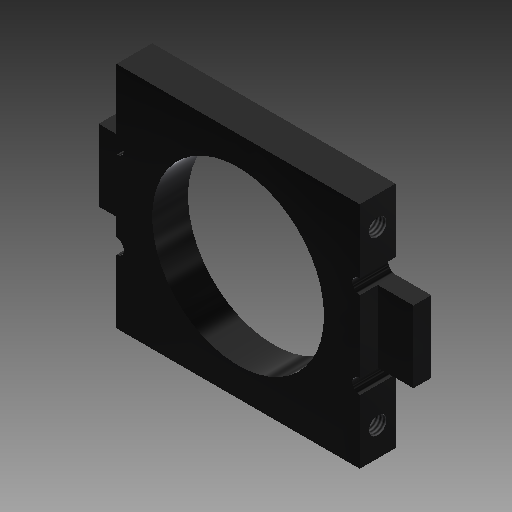
# Autodesk Inventor part: コックピット_2_サブフレーム_6
Saved by Autodesk Inventor 2018 (Build 220112000, 112)
## iProperties
Category: コックピット
Created: 2016-05-24
Part Number: コックピット_2_サブフレーム_6
Material: アセタール樹脂、黒
Document SubType Name: Modeling
Designer: hiroaki
Density: 1.425 g/cm^3
Appearance: 滑らか - 黒
Mass: 4.76795 g
Surface Area: 26.4558 cm^2
Volume: 3.34593 cm^3
Author: hiroaki
Autodesk Inventor part; units mm, degrees
ref_plane "YZ Plane" through (0, 0, 0) normal (1, 0, 0) x (0, 1, 0)
ref_plane "XZ Plane" through (0, 0, 0) normal (0, 1, 0) x (-1, 0, 0)
ref_plane "XY Plane" through (0, 0, 0) normal (0, 0, 1) x (1, 0, 0)
sketch "スケッチ1" plane through (0, 0, 0) normal (0, 0, 1) x (1, 0, 0)
  line L0 (-17, -16) -> (17, -16) construction
  line L1 (17, -16) -> (17, 16) construction
  line L2 (17, 16) -> (-17, 16) construction
  line L3 (-17, 16) -> (-17, -16) construction
  line L4 (-17, -16) -> (17, 16) construction
  line L5 (17, -16) -> (-17, 16) construction
  line L6 (-17, 7.1) -> (-17, 16)
  line L7 (-17, 16) -> (17, 16)
  line L8 (17, 16) -> (17, 7.1)
  line L9 (-17, 5) -> (-22, 5)
  line L10 (-22, 5) -> (-22, -5)
  line L11 (-22, -5) -> (-17, -5)
  line L12 (17, 5) -> (22, 5)
  line L13 (22, 5) -> (22, -5)
  line L14 (22, -5) -> (17, -5)
  line L15 (-17, -7.1) -> (-17, -16)
  line L16 (-17, -16) -> (17, -16)
  line L17 (17, -16) -> (17, -7.1)
  arc A0 (-17, 5) -> (-17, 7.1) centre (-17, 6.05) ccw
  arc A1 (-17, -7.1) -> (-17, -5) centre (-17, -6.05) ccw
  arc A2 (17, 7.1) -> (17, 5) centre (17, 6.05) ccw
  arc A3 (17, -5) -> (17, -7.1) centre (17, -6.05) ccw
  line L18 (0, 0) -> (-17, 0) construction
  line L19 (0, 0) -> (0, 16) construction
  dimension "d87" = 32
  dimension "d88" = 1.05
  dimension "d89" = 5
  dimension "d90" = 11
  dimension "d91" = 34
  constraints: 40 end point, 8 point on circle, 6 collinear, 6 perpendicular, 4 centre point, 4 horizontal, 4 midpoint, 4 point on line, 3 equal radius, 3 parallel, 3 symmetric about line, 2 tangent, 1 vertical, 3 other
  measures "d87" distance of L2.end L0.start
  measures "d88" radius of A0
  measures "d89" distance between parallel lines of L10 L3
  measures "d90" distance between parallel lines of L2 L9
  measures "d91" distance of L1.end L2.end
extrude "押し出し1" add sketch "スケッチ1" along normal blind 5
sketch "スケッチ2" plane through (0, 0, 5) normal (0, 0, 1) x (1, 0, 0)
  line L0 (-17, 16) -> (-17, 7.1) projected
  line L1 (17, 7.1) -> (17, 16) projected
  line L2 (-28.2886, 18.8938) -> (-17, 18.8938)
  line L3 (-17, 18.8938) -> (-17, -23.6662)
  line L4 (-17, -23.6662) -> (-28.2886, -23.6662)
  line L5 (-28.2886, -23.6662) -> (-28.2886, 18.8938)
  line L6 (17, 13.565) -> (34.37, 13.565)
  line L7 (34.37, 13.565) -> (34.37, -20.2305)
  line L8 (34.37, -20.2305) -> (17, -20.2305)
  line L9 (17, -20.2305) -> (17, 13.565)
  point P0 (0, 0)
  constraints: 16 end point, 4 parallel, 2 collinear, 2 horizontal, 2 perpendicular
extrude "押し出し2" cut sketch "スケッチ2" against normal blind 2.5
sketch "スケッチ3" plane through (17, -16, 0) normal (1, 0, 0) x (0, 0, -1)
  line L0 (0, 0) -> (-5, 0) projected
  line L1 (-5, 11) -> (-5, 21) construction
  line L2 (-5, 16) -> (0, 16) construction
  point P0 (-2.5, 4)
  point P1 (-2.5, 28)
  point P2 (-2.5, 0)
  dimension "d96" = 4
  constraints: 2 end point, 2 midpoint, 1 horizontal, 1 symmetric about line, 1 vertical alignment
  measures "d96" distance from line of L0 point (-2.5, 4)
hole "穴1" at (17, -12, 2.5) at (17, 12, 2.5) direction (-1, 0, 0) diameter 2.459 depth 2.5 thread size "M3x0.5" class "6H" standard "ISO Metric profile"
mirror "ミラー1" about plane through (0, 0, 0) normal (1, 0, 0) of "穴1"
sketch "スケッチ4" plane through (0, 0, 5) normal (0, 0, 1) x (1, 0, 0)
  line L0 (-17, -16) -> (17, -16) projected
  line L1 (17, -16) -> (17, -7.1) projected
  line L2 (10, 12) -> (-10, 12) construction
  line L3 (-10, 12) -> (-10, -12) construction
  line L4 (-10, -12) -> (10, -12) construction
  line L5 (10, -12) -> (10, 12) construction
  line L6 (10, 12) -> (-10, -12) construction
  line L7 (-10, 12) -> (10, -12) construction
  circle A0 centre (0, 0) radius 12
  dimension "d104" = 4
  dimension "d105" = 7
  constraints: 12 end point, 2 midpoint, 2 parallel, 1 centre point, 1 coincident, 1 horizontal, 1 perpendicular, 1 tangent
  measures "d104" distance between parallel lines of L0 L4
  measures "d105" distance between parallel lines of L1 L5
extrude "押し出し3" cut sketch "スケッチ4" against normal blind 10
equation "\"d87\" = d3"
equation "\"d90\" = d77 + d82"
equation "\"d96\" = d77"
equation "\"d3\" = 32"
equation "\"d77\" = 4"
equation "\"d82\" = 7"
